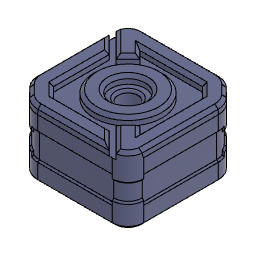
Steppy Unibody (Autodesk Fusion 360 design; units mm, degrees)
Autodesk Fusion 360 part; units mm, degrees
sketch "Sketch1" plane through (0, 0, 0) normal (0, 0, 1) x (1, 0, 0) in component "Frame"
  line L0 (15, 15) -> (-15, 15)
  line L1 (-15, 15) -> (-15, -15)
  line L2 (-15, -15) -> (15, -15)
  line L3 (15, -15) -> (15, 15)
  line L4 (15, 15) -> (-15, -15) construction
  line L5 (-15, 15) -> (15, -15) construction
  circle A0 centre (0, 0) radius 8.6066
  line L6 (9.8361, 15) -> (15, 9.8361)
  line L7 (-15, -9.8361) -> (-9.8361, -15)
  circle A1 centre (0, 0) radius 4.3279
  line L8 (5.7832, -8.8087) -> (8.8087, -5.7832)
  line L9 (8.8087, -5.7832) -> (10.7213, -7.6958)
  line L10 (10.7213, -7.6958) -> (10.7213, 8.0638)
  line L11 (10.7213, 8.0638) -> (8.0638, 10.7213)
  line L12 (8.0638, 10.7213) -> (-7.6958, 10.7213)
  line L13 (-7.6958, 10.7213) -> (-5.7832, 8.8087)
  line L14 (-5.7832, 8.8087) -> (-8.8087, 5.7832)
  line L15 (-8.8087, 5.7832) -> (-15, 11.9745)
  line L16 (5.7832, -8.8087) -> (11.9745, -15)
  line L17 (-15, 10.263) -> (-10.7213, 5.9843)
  line L18 (-10.7213, 5.9843) -> (-10.7213, -8.0638)
  line L19 (-10.7213, -8.0638) -> (-8.0638, -10.7213)
  line L20 (-8.0638, -10.7213) -> (5.9843, -10.7213)
  line L21 (5.9843, -10.7213) -> (10.263, -15)
  point P0 (15, 9.8361)
  point P1 (9.8361, 15)
  point P2 (-7.296, 7.296)
  point P3 (7.296, -7.296)
  point P4 (-6.0858, 6.0858)
  point P5 (6.0858, -6.0858)
  dimension "d2" = 30
  dimension "d3" = 17.2131
  dimension "d4" = 5.1639
  dimension "d5" = 5.1639
  dimension "d6" = 5.1639
  dimension "d7" = 5.1639
  dimension "d8" = 8.6557
  dimension "d10" = 4.2787
  dimension "d11" = 4.2787
  dimension "d12" = 4.2787
  dimension "d13" = 4.2787
  dimension "d15" = 4.2787
  dimension "d16" = 4.2787
  dimension "d17" = 4.2787
  dimension "d18" = 1.7115
  dimension "d19" = 1.7115
  dimension "d20" = 1.7115
  dimension "d21" = 1.7115
  constraint horizontal L0
  constraint perpendicular L0 L1
  constraint parallel L0 L2
  constraint parallel L1 L3
  constraint coincident L4 A0.centre
  constraint coincident L5 A0.centre
  constraint coincident A0.centre A1.centre
  constraint equal L2 L3
  constraint coincident L0 P1
  constraint coincident L3 P0
  constraint coincident P0 L6.end
  constraint coincident P1 L6.start
  constraint coincident L1 L7.start
  constraint coincident L2 L7.end
  constraint perpendicular L5 L8
  constraint perpendicular L8 L9
  constraint vertical L10
  constraint perpendicular L8 L11
  constraint horizontal L12
  constraint parallel L11 L13
  constraint perpendicular L11 L14
  constraint coincident L1 L15.end
  constraint perpendicular L14 L15
  constraint coincident L2 L16.end
  constraint perpendicular L8 L16
  constraint coincident L1 L17.start
  constraint parallel L1 L18
  constraint perpendicular L18 L20
  constraint coincident L2 L21.end
  constraint parallel L7 L19
  constraint parallel L16 L21
  constraint parallel L15 L17
  constraint midpoint L14 P2
  constraint coincident L5 P2
  constraint midpoint L8 P3
  constraint coincident L5 P3
  constraint equal L8 L14
  constraint coincident L5 P4
  constraint coincident A0 P4
  constraint coincident L5 P5
  constraint coincident A0 P5
  measures "d2" distance of L0.start L2.end
  measures "d3" diameter of A0
  measures "d4" distance of L0.start P0
  measures "d5" distance of L0.start L6.start
  measures "d6" distance of L1.end L7.end
  measures "d7" distance of L1.end L7.start
  measures "d8" diameter of A1
  measures "d10" distance of L3 L10
  measures "d11" distance of L6 L11
  measures "d12" distance of L0 L12
  measures "d13" distance of L13.end L14.end
  measures "d15" distance of L2 L20
  measures "d16" distance of L1 L18
  measures "d17" distance of L7 L19
  measures "d18" distance of L16.end L21.end
  measures "d19" distance of L15.end L17.start
  measures "d20" distance of P2 P4
  measures "d21" distance of P3 P5
extrude "Extrude1" add sketch "Sketch1" against normal blind 15 contours L0 L1 L2 L3 L6 L8 L9 L10 L11 L12 L13 L14 L15 L16 | L1 L2 L8 L9 L10 L11 L12 L13 L14 L15 L16 L17 L18 L19 L20 L21 | L1 L2 L7 L17 L18 L19 L20 L21 | A0 | A1 makes body 1 in component "Frame"
extrude "Extrude1'" add sketch "Sketch1" along normal blind 2 draft -1 contours L0 L1 L2 L3 L6 L8 L9 L10 L11 L12 L13 L14 L15 L16 | L1 L2 L7 L17 L18 L19 L20 L21 | A0 bodies 1 in component "Frame"
fillet "Fillet1" radius 5 8 edges at (15, 9.8361, -7.5) (14.9825, 9.8288, 1) (9.8361, 15, -7.5) (9.8288, 14.9825, 1) (-9.8361, -15, -7.5) (-9.8288, -14.9825, 1) (-14.9825, -9.8288, 1) (-15, -9.8361, -7.5) on bodies 1 in component "Frame"
fillet "Fillet1" radius 4 4 edges at (-15, 15, -7.5) (-14.9825, 14.9825, 1) (15, -15, -7.5) (14.9825, -14.9825, 1) on bodies 1 in component "Frame"
hole "Hole1" at (0, 0, 0) direction (0, 0, -1) diameter 5 end through all bodies 1 in component "Frame"
sketch "Sketch2" plane through (0, 0, -15) normal (0, 0, -1) x (1, 0, 0) in component "Frame"
  circle A0 centre (0, 0) radius 2.5
  arc A1 (-15, -11) -> (-11, -15) centre (-11, -11) ccw
  line L0 (-11, -15) -> (7.765, -15)
  arc A2 (7.765, -15) -> (11.3005, -13.5355) centre (7.765, -10) ccw
  line L1 (11.3005, -13.5355) -> (13.5355, -11.3005)
  arc A3 (13.5355, -11.3005) -> (15, -7.765) centre (10, -7.765) ccw
  line L2 (15, -7.765) -> (15, 11)
  arc A4 (15, 11) -> (11, 15) centre (11, 11) ccw
  line L3 (11, 15) -> (-7.765, 15)
  arc A5 (-7.765, 15) -> (-11.3005, 13.5355) centre (-7.765, 10) ccw
  line L4 (-11.3005, 13.5355) -> (-13.5355, 11.3005)
  arc A6 (-13.5355, 11.3005) -> (-15, 7.765) centre (-10, 7.765) ccw
  line L5 (-15, 7.765) -> (-15, -11)
  line L6 (-11.0177, 13.2527) -> (-13.2527, 11.0177)
  arc A7 (-13.2527, 11.0177) -> (-14.6, 7.765) centre (-10, 7.765) ccw
  line L7 (-14.6, 7.765) -> (-14.6, -11)
  arc A8 (-14.6, -11) -> (-11, -14.6) centre (-11, -11) ccw
  line L8 (-11, -14.6) -> (7.765, -14.6)
  arc A9 (7.765, -14.6) -> (11.0177, -13.2527) centre (7.765, -10) ccw
  line L9 (11.0177, -13.2527) -> (13.2527, -11.0177)
  arc A10 (13.2527, -11.0177) -> (14.6, -7.765) centre (10, -7.765) ccw
  line L10 (14.6, -7.765) -> (14.6, 11)
  arc A11 (14.6, 11) -> (11, 14.6) centre (11, 11) ccw
  line L11 (11, 14.6) -> (-7.765, 14.6)
  arc A12 (-7.765, 14.6) -> (-11.0177, 13.2527) centre (-7.765, 10) ccw
  dimension "d31" = -0.4
extrude "Extrude2" cut sketch "Sketch2" against normal up to surface (6 mm away) from surface at -5 contours A1 L0 A2 L1 A3 L2 A4 L3 A5 L4 A6 L5 bodies 1 in component "Frame"
sketch "Sketch1 (2)" plane through (0, 0, 0) normal (0, 0, 1) x (-1, 0, 0) in component "Shaft"
  line L0 (-5.9843, 10.7213) -> (-10.263, 15)
  line L1 (-10.263, 15) -> (-11, 15)
  line L2 (-11.8772, 14.9026) -> (-5.7832, 8.8087)
  line L3 (-5.7832, 8.8087) -> (-8.8087, 5.7832)
  line L4 (-8.8087, 5.7832) -> (-10.7213, 7.6958)
  line L5 (-10.7213, 7.6958) -> (-10.7213, -8.0638)
  line L6 (-10.7213, -8.0638) -> (-8.0638, -10.7213)
  line L7 (-8.0638, -10.7213) -> (7.6958, -10.7213)
  line L8 (7.6958, -10.7213) -> (5.7832, -8.8087)
  line L9 (5.7832, -8.8087) -> (8.8087, -5.7832)
  line L10 (8.8087, -5.7832) -> (14.9026, -11.8772)
  line L11 (15, -11) -> (15, -10.263)
  line L12 (15, -10.263) -> (10.7213, -5.9843)
  line L13 (10.7213, -5.9843) -> (10.7213, 8.0638)
  line L14 (10.7213, 8.0638) -> (8.0638, 10.7213)
  line L15 (8.0638, 10.7213) -> (-5.9843, 10.7213)
  circle A0 centre (0, 0) radius 8.6066
  circle A1 centre (0, 0) radius 2.5
  arc A2 (-11, 15) -> (-11.8772, 14.9026) centre (-11, 11) ccw
  arc A3 (14.9026, -11.8772) -> (15, -11) centre (11, -11) ccw
  dimension "d35" = 5
  constraint concentric A0 A1
  measures "d35" diameter of A1
extrude "Extrude1''" add sketch "Sketch1 (2)" along normal blind 5 and the other way up to surface (13 mm away) separate body contours A1 makes body 2 in component "Shaft"
sketch "Sketch2 (2)" plane through (0, 0, 5) normal (0, 0, 1) x (-1, 0, 0) in component "Shaft"
  circle A0 centre (0, 0) radius 2.5
  line L0 (1.1091, -2.2405) -> (-2.2405, 1.1091)
  line L1 (0, 0) -> (-2.5, 0) construction
  dimension "d40" = 45
  dimension "d41" = 0.8
  constraint coincident A0 L0.start
  constraint coincident A0 L0.end
  constraint coincident A0.centre L1.start
  constraint coincident A0 L1.end
  constraint horizontal L1
  measures "d40" angle of L0 L1
  measures "d41" distance of A0.centre L0
extrude "Extrude2'" cut sketch "Sketch2 (2)" against normal blind 2 contours A0 L0 picked at (-0.8697, -1.1936) bodies 2 in component "Shaft"
sketch "Sketch1 (1)" plane through (0, 0, 0) normal (1, 0, 0) x (0, 1, 0) in component "Frame"
  line L0 (11.1, -2.4) -> (11.1, -7.5)
  line L1 (11.1, -7.5) -> (11.1, -2.4)
  circle A0 centre (10.5, -3.2) radius 0.6
  circle A1 centre (10.5, -4.4) radius 0.6
  line L2 (10.5, -2.4) -> (10.5, -7.5)
  line L3 (10.5, -2.4) -> (11.1, -2.4) construction
  circle A2 centre (10.5, -5.6) radius 0.6
  circle A3 centre (10.5, -6.8) radius 0.6
  dimension "d70" = 1.2
  dimension "d71" = 0.8
  constraint tangent A0 A1
  constraint equal A0 A1
  constraint parallel L1 L2
  constraint coincident L0.start L1.end
  constraint perpendicular L1 L3
  constraint coincident A0.centre L2
  constraint coincident A1.centre L2
  constraint tangent L1 A0
  constraint equal L1 L2
  constraint coincident L2 A2.centre
  constraint tangent A1 A2
  constraint coincident L2 A3.centre
  constraint tangent A2 A3
  constraint equal A1 A2
  constraint equal A2 A3
  measures "d70" diameter of A0
  measures "d71" distance of A0.centre L2.start
sweep "Sweep1" [suppressed] in component "Frame"
sketch "Sketch2 (1)" plane through (0, 0, -15) normal (0, 0, -1) x (1, 0, 0) in component "Frame"
  circle A0 centre (0, 0) radius 2.5
  arc A1 (-15, -11) -> (-11, -15) centre (-11, -11) ccw
  line L0 (-11, -15) -> (7.765, -15)
  arc A2 (7.765, -15) -> (11.3005, -13.5355) centre (7.765, -10) ccw
  line L1 (11.3005, -13.5355) -> (13.5355, -11.3005)
  arc A3 (13.5355, -11.3005) -> (15, -7.765) centre (10, -7.765) ccw
  line L2 (15, -7.765) -> (15, 11)
  arc A4 (15, 11) -> (11, 15) centre (11, 11) ccw
  line L3 (11, 15) -> (-7.765, 15)
  arc A5 (-7.765, 15) -> (-11.3005, 13.5355) centre (-7.765, 10) ccw
  line L4 (-11.3005, 13.5355) -> (-13.5355, 11.3005)
  arc A6 (-13.5355, 11.3005) -> (-15, 7.765) centre (-10, 7.765) ccw
  line L5 (-15, 7.765) -> (-15, -11)
  circle A7 centre (0, 0) radius 1.75
  dimension "d64" = 3.5
  constraint coincident A0.centre A7.centre
  measures "d64" diameter of A7
extrude "Extrude3" add sketch "Sketch2 (1)" against normal up to surface (2 mm away) contours A0 bodies 1 in component "Frame"
chamfer "Chamfer1" distance 0.8 angle 45 41 edges at (-1.6316, -0.6328, -15) (1.6175, -15, -15) (-9.6784, -14.6194, -15) (-12.418, -12.418, -15) (-14.6194, -9.6784, -15) (-15, 1.6175, -15) (-13.8284, 13.8284, -15) (-1.6175, 15, -15) (9.6784, 14.6194, -15) (12.418, 12.418, -15) (14.6194, 9.6784, -15) (15, -1.6175, -15) (13.8284, -13.8284, -15) (-14.9651, 1.214, 2) (-14.5846, -9.664, 2) (-12.3933, -12.3933, 2) (-9.664, -14.5846, 2) (1.214, -14.9651, 2) (-1.8882, 14.9651, 2) (9.664, 14.5846, 2) (12.3933, 12.3933, 2) (14.5846, 9.664, 2) (14.9651, -1.8882, 2) (8.0743, -12.8607, 2) (-1.0542, -10.7562, 2) (-9.4172, -9.4172, 2) (-10.7562, -1.0542, 2) (-12.8607, 8.0743, 2) (8.8749, -11.851, 2) (7.3206, -7.3206, 2) (9.7825, -6.8063, 2) (10.7562, 0.1491, 2) (9.4172, 9.4172, 2) (0.1491, 10.7562, 2) (-6.8063, 9.7825, 2) (-7.3206, 7.3206, 2) (-11.851, 8.8749, 2) (-7.9916, 3.0996, 2) (-4.0675, 1.5776, 2) (13.9651, -13.6848, 2) (-13.6848, 13.9651, 2) on bodies 1 in component "Frame"
sketch "Sketch3" plane through (0, 0, -10) normal (0, 0, 1) x (-1, 0, 0) in component "Frame"
  arc A0 (11.0177, 13.2527) -> (7.765, 14.6) centre (7.765, 10) ccw
  line L0 (11.0177, 13.2527) -> (13.2527, 11.0177)
  arc A1 (14.6, 7.765) -> (13.2527, 11.0177) centre (10, 7.765) ccw
  line L1 (14.6, 7.765) -> (14.6, -11)
  arc A2 (11, -14.6) -> (14.6, -11) centre (11, -11) ccw
  line L2 (11, -14.6) -> (-7.765, -14.6)
  arc A3 (-11.0177, -13.2527) -> (-7.765, -14.6) centre (-7.765, -10) ccw
  line L3 (-11.0177, -13.2527) -> (-13.2527, -11.0177)
  arc A4 (-14.6, -7.765) -> (-13.2527, -11.0177) centre (-10, -7.765) ccw
  line L4 (-14.6, -7.765) -> (-14.6, 11)
  arc A5 (-11, 14.6) -> (-14.6, 11) centre (-11, 11) ccw
  line L5 (-11, 14.6) -> (7.765, 14.6)
  line L6 (15, -11) -> (15, 7.765)
  arc A6 (15, 7.765) -> (13.5355, 11.3005) centre (10, 7.765) ccw
  line L7 (13.5355, 11.3005) -> (11.3005, 13.5355)
  arc A7 (11.3005, 13.5355) -> (7.765, 15) centre (7.765, 10) ccw
  line L8 (7.765, 15) -> (-11, 15)
  arc A8 (-11, 15) -> (-15, 11) centre (-11, 11) ccw
  line L9 (-15, 11) -> (-15, -7.765)
  arc A9 (-15, -7.765) -> (-13.5355, -11.3005) centre (-10, -7.765) ccw
  line L10 (-13.5355, -11.3005) -> (-11.3005, -13.5355)
  arc A10 (-11.3005, -13.5355) -> (-7.765, -15) centre (-7.765, -10) ccw
  line L11 (-7.765, -15) -> (11, -15)
  arc A11 (11, -15) -> (15, -11) centre (11, -11) ccw
  line L12 (14.6194, 9.6784) -> (14.2498, 9.5253)
  line L13 (9.6784, 14.6194) -> (9.5253, 14.2498)
  line L14 (-11, 15) -> (-11, 14.6)
  line L15 (-15, 11) -> (-14.6, 11)
  line L16 (-14.6194, -9.6784) -> (-14.2498, -9.5253)
  line L17 (-9.6784, -14.6194) -> (-9.5253, -14.2498)
  line L18 (11, -15) -> (11, -14.6)
  line L19 (15, -11) -> (14.6, -11)
  constraint midpoint A6 L12.start
  constraint midpoint A1 L12.end
  constraint coincident A7 L13.start
  constraint coincident A0 L13.end
  constraint midpoint A7 L13.start
  constraint midpoint A0 L13.end
  constraint coincident L8.end A8.start
  constraint coincident A5.start L5.start
  constraint coincident A8.end L9.start
  constraint coincident L4.end A5.end
  constraint midpoint A9 L16.start
  constraint midpoint A4 L16.end
  constraint midpoint A10 L17.start
  constraint midpoint A3 L17.end
  constraint coincident L11.end A11.start
  constraint coincident A2.start L2.start
  constraint coincident L6.start A11.end
  constraint coincident L1.end A2.end
extrude "Extrude4" add sketch "Sketch3" along normal blind 1 contours A0 L0 A1 A6 L7 A7 L12 L13 | A5 A8 L14 L15 | A2 A11 L18 L19 | A3 L3 A4 A9 L10 A10 L16 L17 bodies 1 in component "Frame"
sketch "Sketch4" plane through (0, 0, -4) normal (0, 0, -1) x (1, 0, 0) in component "Frame"
  line L0 (-7.765, 14.6) -> (11, 14.6)
  arc A0 (14.6, 11) -> (11, 14.6) centre (11, 11) ccw
  line L1 (14.6, 11) -> (14.6, -7.765)
  arc A1 (13.2527, -11.0177) -> (14.6, -7.765) centre (10, -7.765) ccw
  line L2 (13.2527, -11.0177) -> (11.0177, -13.2527)
  arc A2 (7.765, -14.6) -> (11.0177, -13.2527) centre (7.765, -10) ccw
  line L3 (7.765, -14.6) -> (-11, -14.6)
  arc A3 (-14.6, -11) -> (-11, -14.6) centre (-11, -11) ccw
  line L4 (-14.6, -11) -> (-14.6, 7.765)
  arc A4 (-13.2527, 11.0177) -> (-14.6, 7.765) centre (-10, 7.765) ccw
  line L5 (-13.2527, 11.0177) -> (-11.0177, 13.2527)
  arc A5 (-7.765, 14.6) -> (-11.0177, 13.2527) centre (-7.765, 10) ccw
  arc A6 (-15, -11) -> (-11, -15) centre (-11, -11) ccw
  line L6 (-11, -15) -> (7.765, -15)
  arc A7 (7.765, -15) -> (11.3005, -13.5355) centre (7.765, -10) ccw
  line L7 (11.3005, -13.5355) -> (13.5355, -11.3005)
  arc A8 (13.5355, -11.3005) -> (15, -7.765) centre (10, -7.765) ccw
  line L8 (15, -7.765) -> (15, 11)
  arc A9 (15, 11) -> (11, 15) centre (11, 11) ccw
  line L9 (11, 15) -> (-7.765, 15)
  arc A10 (-7.765, 15) -> (-11.3005, 13.5355) centre (-7.765, 10) ccw
  line L10 (-11.3005, 13.5355) -> (-13.5355, 11.3005)
  arc A11 (-13.5355, 11.3005) -> (-15, 7.765) centre (-10, 7.765) ccw
  line L11 (-15, 7.765) -> (-15, -11)
  line L12 (11, 14.6) -> (11, 15)
  line L13 (14.6, 11) -> (15, 11)
  line L14 (-9.5253, 14.2498) -> (-9.6784, 14.6194)
  line L15 (-14.2498, 9.5253) -> (-14.6194, 9.6784)
  line L16 (-14.6, -11) -> (-15, -11)
  line L17 (-11, -14.6) -> (-11, -15)
  line L18 (9.6784, -14.6194) -> (9.5253, -14.2498)
  line L19 (14.6194, -9.6784) -> (14.2498, -9.5253)
  constraint coincident L0.end A0.end
  constraint coincident A9.end L9.start
  constraint coincident A0.start L1.start
  constraint coincident L8.end A9.start
  constraint midpoint A5 L14.start
  constraint midpoint A10 L14.end
  constraint midpoint A4 L15.start
  constraint midpoint A11 L15.end
  constraint coincident A3.start L4.start
  constraint coincident A6.start L11.end
  constraint coincident L3.end A3.end
  constraint coincident A6.end L6.start
  constraint midpoint A7 L18.start
  constraint midpoint A2 L18.end
  constraint midpoint A8 L19.start
  constraint midpoint A1 L19.end
extrude "Extrude5" add sketch "Sketch4" along normal blind 1 contours A0 A9 L12 L13 | A4 L5 A5 A10 L10 A11 L14 L15 | A1 L2 A2 A7 L7 A8 L18 L19 | A3 A6 L16 L17 bodies 1 in component "Frame"
chamfer "Chamfer2" distance 0.4 angle 45 32 edges at (12.418, 12.418, -5) (14.1573, 10.5428, -5) (10.5428, 14.1573, -5) (13.8284, -13.8284, -5) (15, -1.6175, -4) (14.9039, 8.7404, -4) (1.6175, -15, -4) (-8.7404, -14.9039, -4) (-10.5428, -14.1573, -5) (-12.418, -12.418, -5) (-14.1573, -10.5428, -5) (-15, 1.6175, -4) (-14.9039, -8.7404, -4) (-13.8284, 13.8284, -5) (-1.6175, 15, -4) (8.7404, 14.9039, -4) (-1.6175, 15, -10) (8.7404, 14.9039, -10) (-13.8284, 13.8284, -9) (12.418, 12.418, -9) (10.5428, 14.1573, -9) (14.1573, 10.5428, -9) (14.9039, 8.7404, -10) (15, -1.6175, -10) (13.8284, -13.8284, -9) (1.6175, -15, -10) (-8.7404, -14.9039, -10) (-12.418, -12.418, -9) (-10.5428, -14.1573, -9) (-14.1573, -10.5428, -9) (-15, 1.6175, -10) (-14.9039, -8.7404, -10) on bodies 1 in component "Frame"
chamfer "Chamfer1'" distance 0.5 angle 45 1 edges at (-1.7678, -1.7678, 5) on bodies 2 in component "Shaft"
ref_plane "WorkPlane1" through (0, 0, 12.125) normal (0.707107, 0.707107, 0) x (0, 0, 1) in component "Frame"
sketch "Sketch5" plane through (0, 0, 12.125) normal (0.707107, 0.707107, 0) x (0, 0, 1) in component "Frame"
  line L0 (-27.125, 2.55) -> (-27.125, -2.55)
  line L1 (-27.125, 17.8191) -> (-27.125, 4.5502)
  line L2 (-27.125, 1.5804) -> (-27.125, 4.5502)
  line L3 (-27.125, 1.5804) -> (-27.125, -1.5804)
  line L4 (-27.125, -4.5502) -> (-27.125, -1.5804)
  line L5 (-27.125, -4.5502) -> (-27.125, -17.8191)
  line L6 (-27.125, -18.7563) -> (-27.125, -17.8191)
  line L7 (-27.125, -17.8191) -> (-27.125, -4.5502)
  line L8 (-27.125, -4.5502) -> (-27.125, -1.5804)
  line L9 (-27.125, -1.5804) -> (-27.125, 1.5804)
  line L10 (-27.125, 1.5804) -> (-27.125, 4.5502)
  line L11 (-27.125, 4.5502) -> (-27.125, 17.8191)
  line L12 (-27.125, 17.8191) -> (-27.125, 18.7563)
  line L13 (-21.525, 18.3848) -> (-21.525, 19.5563)
  line L14 (-21.525, 18.3848) -> (-22.525, 18.3848)
  line L15 (-22.525, 18.3848) -> (-26.325, 18.3848)
  line L16 (-26.325, 19.5563) -> (-26.325, 18.3848)
  line L17 (-26.325, 18.3848) -> (-22.525, 18.3848)
  line L18 (-22.525, 18.3848) -> (-21.525, 18.3848)
  line L19 (-27.125, 11.1847) -> (-25.925, 11.1847)
  line L20 (-25.925, 13.6847) -> (-25.925, 8.6847)
  line L21 (-25.925, 13.6847) -> (-27.125, 13.6847)
  line L22 (-25.925, 8.6847) -> (-27.125, 8.6847)
  line L23 (-27.125, 15.6847) -> (-23.925, 15.6847)
  line L24 (-23.925, 15.6847) -> (-23.925, 6.6847)
  line L25 (-23.925, 6.6847) -> (-27.125, 6.6847)
  line L26 (-25.525, 15.6847) -> (-23.925, 14.0847)
  line L27 (-23.925, 8.2847) -> (-25.525, 6.6847)
  dimension "d80" = 1.2
  dimension "d81" = 5
  dimension "d82" = 2
  dimension "d83" = 2
  dimension "d84" = 2
  dimension "d85" = 45
  dimension "d86" = 45
  constraint midpoint L11 L19.start
  constraint perpendicular L1 L19
  constraint vertical L20
  constraint midpoint L19.end L20
  constraint coincident L1 L21.end
  constraint perpendicular L1 L21
  constraint coincident L11 L22.end
  constraint perpendicular L11 L22
  constraint coincident L11 L23.start
  constraint perpendicular L1 L23
  constraint perpendicular L23 L24
  constraint coincident L11 L25.end
  constraint perpendicular L11 L25
  constraint coincident L23 L26.start
  constraint coincident L24 L26.end
  constraint coincident L24 L27.start
  constraint midpoint L25 L27.end
  constraint midpoint L23 L26.start
  measures "d80" distance of L19.start L19.end
  measures "d81" distance of L20.start L20.end
  measures "d82" distance of L21.end L23.start
  measures "d83" distance of L22.end L25.end
  measures "d84" distance of L20 L24
  measures "d85" angle of L23 L26
  measures "d86" angle of L25 L27
extrude "Extrude6" cut sketch "Sketch5" along normal mid plane 4 contours L1 L11 L20 L21 L22 L23 L24 L25 L26 L27 bodies 1 in component "Frame"
fillet "Fillet2" radius 0.6 1 edges at (-2.3308, 0.904, 0) on bodies 1 in component "Frame"
component "Frame" placed x (1, 0, 0) y (0, 1, 0) z (0, 0, 1) at (0, 0, 0)
component "Shaft" placed x (1, 0, 0) y (0, 1, 0) z (0, 0, 1) at (0, 0, 0)
equation "FrameSize = 30 mm"
equation "d2 = FrameSize"
equation "d3 = FrameSize * 35 / 61"
equation "d4 = FrameSize * 10.5 / 61"
equation "d5 = FrameSize * 10.5 / 61"
equation "d6 = FrameSize * 10.5 / 61"
equation "d7 = FrameSize * 10.5 / 61"
equation "d8 = FrameSize * 17.6 / 61"
equation "LogoThickness = FrameSize * 8.7 / 61"
equation "d10 = LogoThickness"
equation "d11 = LogoThickness"
equation "d12 = LogoThickness"
equation "d13 = LogoThickness"
equation "d15 = LogoThickness"
equation "d16 = LogoThickness"
equation "d17 = LogoThickness"
equation "d18 = LogoThickness / 2.5"
equation "d19 = LogoThickness / 2.5"
equation "d20 = LogoThickness / 2.5"
equation "d21 = LogoThickness / 2.5"
equation "d22 = -FrameSize * 2 / 4"
